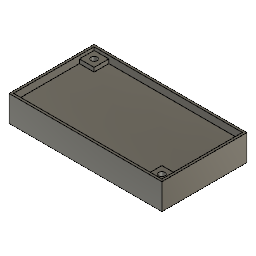
Bas (Autodesk Fusion 360 design; units mm, degrees)
Autodesk Fusion 360 part; units mm, degrees
sketch "Sketch2" plane through (0, 0, 0) normal (0, 0, 1) x (1, 0, 0)
  line L0 (0, 0) -> (79, 0)
  line L1 (79, 0) -> (79, 44)
  line L2 (79, 44) -> (0, 44)
  line L3 (0, 44) -> (0, 0)
  line L4 (1.2, 1.2) -> (77.8, 1.2)
  line L5 (77.8, 1.2) -> (77.8, 42.8)
  line L6 (77.8, 42.8) -> (1.2, 42.8)
  line L7 (1.2, 42.8) -> (1.2, 1.2)
  circle A0 centre (5, 39) radius 1.6
  line L8 (6.5877, 41.75) -> (3.4123, 41.75)
  line L9 (3.4123, 41.75) -> (1.8246, 39)
  line L10 (1.8246, 39) -> (3.4123, 36.25)
  line L11 (3.4123, 36.25) -> (6.5877, 36.25)
  line L12 (6.5877, 36.25) -> (8.1754, 39)
  line L13 (8.1754, 39) -> (6.5877, 41.75)
  line L14 (2, 2) -> (77, 2)
  line L15 (77, 2) -> (77, 42)
  line L16 (77, 42) -> (2, 42)
  line L17 (2, 42) -> (2, 2)
  line L18 (3.4, 41.75) -> (3.4, 36.25)
  line L19 (6.6, 41.75) -> (6.6, 36.25)
  line L20 (3.4, 40.6) -> (6.6, 40.6)
  line L21 (3.4, 37.4) -> (6.6, 37.4)
  circle A1 centre (74, 5) radius 1.6
  line L22 (75.5877, 7.75) -> (72.4123, 7.75)
  line L23 (72.4123, 7.75) -> (70.8246, 5)
  line L24 (70.8246, 5) -> (72.4123, 2.25)
  line L25 (72.4123, 2.25) -> (75.5877, 2.25)
  line L26 (75.5877, 2.25) -> (77.1754, 5)
  line L27 (77.1754, 5) -> (75.5877, 7.75)
  line L28 (72.4, 7.75) -> (72.4, 2.25)
  line L29 (75.6, 7.75) -> (75.6, 2.25)
  line L30 (71.7483, 6.6) -> (76.2517, 6.6)
  line L31 (71.7483, 3.4) -> (76.2517, 3.4)
  point P0 (5, 39)
  point P1 (74, 5)
  dimension "d48" = 44
  dimension "d49" = 79
  dimension "d50" = -1.2
  dimension "d55" = 3.2
  dimension "d56" = 3.8
  dimension "d57" = 3.8
  dimension "d58" = 2.75
  dimension "d59" = -2
  dimension "d60" = 3.2
  dimension "d61" = 3
  dimension "d62" = 3
  dimension "d63" = 2.75
  constraint horizontal L0
  constraint vertical L1
  constraint horizontal L2
  constraint vertical L3
  constraint coincident L0.start L3.end
  constraint coincident P0 A0.centre
  constraint horizontal L8
  constraint coincident L8 L18.start
  constraint coincident L11 L18.end
  constraint perpendicular L11 L18
  constraint coincident L8 L19.start
  constraint coincident L11 L19.end
  constraint perpendicular L11 L19
  constraint tangent A0 L18
  constraint tangent A0 L19
  constraint coincident L18 L20.start
  constraint coincident L19 L20.end
  constraint perpendicular L19 L20
  constraint coincident L18 L21.start
  constraint coincident L19 L21.end
  constraint perpendicular L19 L21
  constraint tangent A0 L20
  constraint tangent A0 L21
  constraint coincident P1 A1.centre
  constraint horizontal L22
  constraint coincident L22 L28.start
  constraint coincident L25 L28.end
  constraint perpendicular L25 L28
  constraint coincident L22 L29.start
  constraint coincident L25 L29.end
  constraint perpendicular L25 L29
  constraint coincident L23 L30.start
  constraint coincident L27 L30.end
  constraint perpendicular L29 L30
  constraint coincident L24 L31.start
  constraint coincident L26 L31.end
  constraint parallel L14 L31
  constraint tangent A1 L28
  constraint tangent A1 L30
  constraint tangent A1 L29
  constraint tangent A1 L31
  measures "d48" distance of L0 L2
  measures "d49" distance of L1 L3
  measures "d55" diameter of A0
  measures "d56" distance of L6 P0
  measures "d57" distance of L7 P0
  measures "d58" distance of P0 L13
  measures "d60" diameter of A1
  measures "d61" distance of L15 P1
  measures "d62" distance of L14 P1
  measures "d63" distance of P1 L27
extrude "Extrude10" add sketch "Sketch2" along normal blind 13.5 contours L0 L1 L2 L3
extrude "Extrude11" add sketch "Sketch2" along normal blind 9.8 contours L4 L5 L6 L7 | A0 | A0 L19 L21 | A0 L19 L20 | L12 L13 L19 | A0 L18 L20 | L8 L9 L13 L18 L19 L20 | A0 L18 L21 | L10 L11 L12 L18 L19 L21 | L9 L10 L17 L18 | L8 L9 L10 L11 L12 L13 L14 L15 L16 L17 L22 L23 L24 L25 L26 L27 | L9 L10 L17 | L15 L26 L27 | L15 L26 L27 L29 L30 L31 | L27 L29 L30 | L26 L29 L31 | L22 L23 L27 L28 L29 L30 | A1 L29 L30 | L24 L25 L26 L28 L29 L31 | A1 L29 L31 | A1 | A1 L28 L30 | A1 L28 L31 | L23 L24 L28 L30 L31 | L23 L28 L30 | L24 L28 L31
ref_plane "WorkPlane2" through (39.5, 22, 9.5) normal (0, 0, 1) x (1, 0, 0)
sketch "Sketch4" plane through (0, 0, 9.5) normal (0, 0, 1) x (1, 0, 0)
  line L0 (3.4, 41.75) -> (3.4, 36.25)
  line L1 (6.5877, 41.75) -> (3.4123, 41.75)
  line L2 (3.4, 40.6) -> (6.6, 40.6)
  line L3 (3.4123, 41.75) -> (1.8246, 39)
  line L4 (1.8246, 39) -> (3.4123, 36.25)
  circle A0 centre (5, 39) radius 1.6
  line L5 (3.4, 37.4) -> (6.6, 37.4)
  line L6 (3.4123, 36.25) -> (6.5877, 36.25)
  line L7 (6.6, 41.75) -> (6.6, 36.25)
  line L8 (8.1754, 39) -> (6.5877, 41.75)
  line L9 (6.5877, 36.25) -> (8.1754, 39)
  line L10 (75.5877, 7.75) -> (72.4123, 7.75)
  line L11 (72.4, 7.75) -> (72.4, 2.25)
  line L12 (71.7483, 6.6) -> (76.2517, 6.6)
  line L13 (72.4123, 7.75) -> (70.8246, 5)
  line L14 (70.8246, 5) -> (72.4123, 2.25)
  line L15 (71.7483, 3.4) -> (76.2517, 3.4)
  circle A1 centre (74, 5) radius 1.6
  line L16 (72.4123, 2.25) -> (75.5877, 2.25)
  line L17 (75.6, 7.75) -> (75.6, 2.25)
  line L18 (77.1754, 5) -> (75.5877, 7.75)
  line L19 (75.5877, 2.25) -> (77.1754, 5)
  line L20 (2, 42) -> (2, 2)
  line L21 (77, 42) -> (2, 42)
  line L22 (2, 2) -> (77, 2)
  line L23 (77, 2) -> (77, 42)
  line L24 (77.8, 42.8) -> (1.2, 42.8)
  line L25 (77.8, 1.2) -> (77.8, 42.8)
  line L26 (1.2, 1.2) -> (77.8, 1.2)
  line L27 (1.2, 42.8) -> (1.2, 1.2)
  line L28 (0, 0) -> (79, 0)
  line L29 (0, 44) -> (0, 0)
  line L30 (79, 0) -> (79, 44)
  line L31 (79, 44) -> (0, 44)
  line L32 (1.2, 42.8) -> (8.8, 42.8)
  line L33 (8.8, 42.8) -> (8.8, 35.2)
  line L34 (8.8, 35.2) -> (1.2, 35.2)
  line L35 (1.2, 35.2) -> (1.2, 42.8)
  line L36 (77.8, 1.2) -> (70.2, 1.2)
  line L37 (70.2, 1.2) -> (70.2, 8.8)
  line L38 (70.2, 8.8) -> (77.8, 8.8)
  line L39 (77.8, 8.8) -> (77.8, 1.2)
  dimension "d90" = 7.6
  dimension "d91" = 7.6
  dimension "d92" = 7.6
  dimension "d93" = 7.6
  constraint horizontal L32
  constraint vertical L33
  constraint horizontal L34
  constraint vertical L35
  constraint coincident L24.end L27.start
  constraint horizontal L36
  constraint vertical L37
  constraint horizontal L38
  constraint vertical L39
  constraint coincident L25.start L26.end
  measures "d90" distance of L24.end L34.end
  measures "d91" distance of L33 L35
  measures "d92" distance of L25.start L38.end
  measures "d93" distance of L37 L39
extrude "Extrude12" cut sketch "Sketch2" along normal blind 14 contours A0
extrude "Extrude13" cut sketch "Sketch2" along normal blind 8.7 contours A0 L19 L21 | A0 L19 L20 | A0 L18 L20 | A0 L18 L21
extrude "Extrude14" cut sketch "Sketch2" along normal blind 8.4 contours L8 L9 L13 L18 L19 L20 | L10 L11 L12 L18 L19 L21
extrude "Extrude15" cut sketch "Sketch2" along normal blind 8.1 contours L12 L13 L19 | L9 L10 L17 L18
extrude "Extrude16" cut sketch "Sketch2" along normal blind 8.1 contours L9 L10 L17
extrude "Extrude17" cut sketch "Sketch2" along normal blind 8.1 contours L15 L26 L27 | L15 L26 L27 L29 L30 L31 | L27 L29 L30 | L26 L29 L31 | L23 L24 L28 L30 L31 | L23 L28 L30 | L24 L28 L31
extrude "Extrude18" cut sketch "Sketch2" along normal blind 8.4 contours L22 L23 L27 L28 L29 L30 | L24 L25 L26 L28 L29 L31
extrude "Extrude19" cut sketch "Sketch2" along normal blind 8.7 contours A1 L29 L30 | A1 L29 L31 | A1 L28 L30 | A1 L28 L31
extrude "Extrude20" cut sketch "Sketch2" along normal blind 14 contours A1
ref_plane "WorkPlane3" through (39.5, 22, 9.8) normal (0, 0, 1) x (1, 0, 0)
sketch "Sketch5" plane through (0, 0, 9.8) normal (0, 0, 1) x (1, 0, 0)
  line L0 (70.2, 8.8) -> (77.8, 8.8)
  line L1 (70.2, 1.2) -> (70.2, 8.8)
  line L2 (77.8, 1.2) -> (70.2, 1.2)
  line L3 (77.8, 8.8) -> (77.8, 1.2)
  line L4 (8.8, 35.2) -> (1.2, 35.2)
  line L5 (8.8, 42.8) -> (8.8, 35.2)
  line L6 (1.2, 35.2) -> (1.2, 42.8)
  line L7 (1.2, 42.8) -> (8.8, 42.8)
  circle A0 centre (5, 39) radius 1.6
  circle A1 centre (74, 5) radius 1.6
extrude "Extrude22" add sketch "Sketch5" along normal blind 2.1 contours L4 L5 L6 L7
extrude "Extrude23" add sketch "Sketch5" along normal blind 2.1 contours L0 L1 L2 L3
